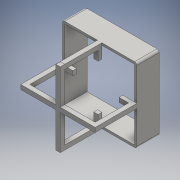
# Autodesk Inventor part: bottom
Saved by Autodesk Inventor 2016 (Build 200138000, 138)
## iProperties
Created: 2015-11-09
Part Number: bottom
Material: Generic
Document SubType Name: Modeling
Designer: Sudhar
Density: 1 g/cm^3
Appearance: Default
Author: Sudhar
Autodesk Inventor part; units mm, degrees
ref_plane "YZ Plane" through (0, 0, 0) normal (1, 0, 0) x (0, 1, 0)
ref_plane "XZ Plane" through (0, 0, 0) normal (0, 1, 0) x (-1, 0, 0)
ref_plane "XY Plane" through (0, 0, 0) normal (0, 0, 1) x (1, 0, 0)
sketch "Sketch1" plane through (0, 0, 0) normal (0, 1, 0) x (-1, 0, 0)
  line L0 (37.3809, 48.8889) -> (-62.6191, 48.8889)
  line L1 (-62.6191, 48.8889) -> (-62.6191, -51.1111)
  line L2 (-62.6191, -51.1111) -> (37.3809, -51.1111)
  line L3 (37.3809, -51.1111) -> (37.3809, 48.8889)
  point P0 (0, 0)
  dimension "d0" = 100
  dimension "d1" = 100
  constraints: 8 end point, 2 parallel, 1 horizontal, 1 perpendicular
  measures "d0" distance of L2.end L0.start
  measures "d1" distance of L1.end L2.end
extrude "Extrusion1" add sketch "Sketch1" along normal blind 30
fillet "Fillet1" radius 3 4 edges at (-37.3809, 15, -51.1111) (-37.3809, 15, 48.8889) (62.6191, 15, -51.1111) (62.6191, 15, 48.8889)
shell "Shell1" thickness 3 removed faces 2 at (27.2857, 30, 14.5556) at (27.2857, 0, 14.5556)
sketch "Sketch2" plane through (0, 0, 0) normal (0, -1, 0) x (1, 0, 0)
  line L0 (-34.3809, 48.8889) -> (59.6191, 48.8889) projected
  line L1 (15.6191, 48.8889) -> (9.6191, 48.8889)
  line L2 (9.6191, 48.8889) -> (9.6191, 29.8889)
  line L3 (9.6191, 29.8889) -> (15.6191, 29.8889)
  line L4 (15.6191, 29.8889) -> (15.6191, 48.8889)
  line L5 (62.6191, 45.8889) -> (62.6191, -48.1111) projected
  line L6 (62.6191, 1.8889) -> (43.6191, 1.8889)
  line L7 (43.6191, 1.8889) -> (43.6191, -4.1111)
  line L8 (43.6191, -4.1111) -> (62.6191, -4.1111)
  line L9 (62.6191, -4.1111) -> (62.6191, 1.8889)
  line L10 (59.6191, -51.1111) -> (-34.3809, -51.1111) projected
  line L11 (15.6191, -32.1111) -> (9.6191, -32.1111)
  line L12 (9.6191, -32.1111) -> (9.6191, -51.1111)
  line L13 (9.6191, -51.1111) -> (15.6191, -51.1111)
  line L14 (15.6191, -51.1111) -> (15.6191, -32.1111)
  line L15 (-37.3809, -48.1111) -> (-37.3809, 45.8889) projected
  line L16 (-18.3809, 1.8889) -> (-37.3809, 1.8889)
  line L17 (-37.3809, 1.8889) -> (-37.3809, -4.1111)
  line L18 (-37.3809, -4.1111) -> (-18.3809, -4.1111)
  line L19 (-18.3809, -4.1111) -> (-18.3809, 1.8889)
  point P0 (0, 0)
  dimension "d6" = 6
  dimension "d7" = 47
  dimension "d8" = 19
  dimension "d9" = 6
  dimension "d10" = 19
  dimension "d11" = 47
  dimension "d12" = 6
  dimension "d13" = 19
  dimension "d14" = 47
  dimension "d15" = 6
  dimension "d16" = 19
  dimension "d17" = 47
  constraints: 32 end point, 8 parallel, 4 horizontal, 4 perpendicular, 4 point on line
  measures "d6" distance of L2.end L3.end
  measures "d7" distance between parallel lines of L4 L5
  measures "d8" distance of L1.end L2.end
  measures "d9" distance of L6.end L7.end
  measures "d10" distance of L7.end L8.end
  measures "d11" distance between parallel lines of L6 L0
  measures "d12" distance of L11.start L11.end
  measures "d13" distance of L13.end L11.start
  measures "d14" distance between parallel lines of L14 L5
  measures "d15" distance of L18.end L16.start
  measures "d16" distance of L17.end L18.end
  measures "d17" distance between parallel lines of L16 L0
extrude "Extrusion2" add sketch "Sketch2" along normal blind 5
sketch "Sketch3" plane through (0, -5, 0) normal (0, -1, 0) x (1, 0, 0)
  line L0 (-34.3809, 48.8889) -> (9.6191, 48.8889) projected
  line L1 (15.6191, 29.8889) -> (15.6191, 45.8889) projected
  line L2 (9.6191, 48.8889) -> (15.6191, 48.8889)
  line L3 (15.6191, 48.8889) -> (15.6191, 42.8889)
  line L4 (15.6191, 42.8889) -> (9.6191, 42.8889)
  line L5 (9.6191, 42.8889) -> (9.6191, 48.8889)
  line L6 (-18.3809, 1.8889) -> (-37.3809, 1.8889) projected
  line L7 (-34.3809, -4.1111) -> (-18.3809, -4.1111) projected
  line L8 (-37.3809, 1.8889) -> (-31.3809, 1.8889)
  line L9 (-31.3809, 1.8889) -> (-31.3809, -4.1111)
  line L10 (-31.3809, -4.1111) -> (-37.3809, -4.1111)
  line L11 (-37.3809, -4.1111) -> (-37.3809, 1.8889)
  line L12 (9.6191, -32.1111) -> (9.6191, -51.1111) projected
  line L13 (9.6191, -45.1111) -> (15.6191, -45.1111)
  line L14 (15.6191, -45.1111) -> (15.6191, -51.1111)
  line L15 (15.6191, -51.1111) -> (9.6191, -51.1111)
  line L16 (9.6191, -51.1111) -> (9.6191, -45.1111)
  line L17 (59.6191, 1.8889) -> (43.6191, 1.8889) projected
  line L18 (62.6191, 45.8889) -> (62.6191, -48.1111) projected
  line L19 (56.6191, 1.8889) -> (62.6191, 1.8889)
  line L20 (62.6191, 1.8889) -> (62.6191, -4.1111)
  line L21 (62.6191, -4.1111) -> (56.6191, -4.1111)
  line L22 (56.6191, -4.1111) -> (56.6191, 1.8889)
  point P0 (0, 0)
  dimension "d20" = 6
  dimension "d21" = 6
  dimension "d22" = 6
  dimension "d23" = 6
  dimension "d24" = 6
  constraints: 32 end point, 8 parallel, 7 point on line, 4 horizontal, 4 perpendicular
  measures "d20" distance of L2.end L3.end
  measures "d21" distance of L3.end L4.end
  measures "d22" distance of L9.end L10.end
  measures "d23" distance of L13.end L14.end
  measures "d24" distance of L20.end L21.end
extrude "Extrusion3" add sketch "Sketch3" along normal blind 45
sketch "Sketch4" plane through (0, -50, 0) normal (0, -1, 0) x (1, 0, 0)
  line L0 (15.6191, -48.1111) -> (15.6191, -51.1111) projected
  line L1 (9.7564, 48.8742) -> (15.6191, 48.8742)
  line L2 (15.6191, -51.1111) -> (9.7564, -51.1111)
  line L3 (-37.3809, 1.8889) -> (-37.3809, 45.8889) projected
  line L4 (62.6191, 45.8889) -> (62.6191, -48.1111) projected
  line L5 (62.6191, 1.8889) -> (62.6191, -4.1419)
  line L6 (-37.3809, -4.1419) -> (-37.3809, 1.8889)
  line L7 (-37.3809, 1.8889) -> (9.7564, 1.8889)
  line L8 (15.6191, 1.8889) -> (62.6191, 1.8889)
  line L9 (9.7564, -51.1111) -> (9.7564, -4.1419)
  line L10 (9.7564, 1.8889) -> (9.7564, 48.8742)
  line L11 (62.6191, -4.1419) -> (15.6191, -4.1419)
  line L12 (9.7564, -4.1419) -> (-37.3809, -4.1419)
  line L13 (15.6191, 48.8742) -> (15.6191, 1.8889)
  line L14 (15.6191, -4.1419) -> (15.6191, -51.1111)
  point P0 (0, 0)
  constraints: 24 end point, 10 parallel, 4 perpendicular, 3 horizontal, 1 point on line
extrude "Extrusion4" add sketch "Sketch4" along normal blind 6
body "Solid1"
